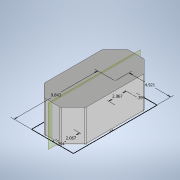
# Autodesk Inventor part: Bottle Holder
Saved by Autodesk Inventor 2020 (Build 240168000, 168)
## iProperties
Created: 2022-01-25
Part Number: Bottle Holder
Material: Generic
Document SubType Name: Modeling
Designer: Beaucage
Density: 1 g/cm^3
Appearance: Default
Author: Beaucage
Autodesk Inventor part; units mm, degrees
ref_plane "YZ Plane" through (0, 0, 0) normal (1, 0, 0) x (0, 1, 0)
ref_plane "XZ Plane" through (0, 0, 0) normal (0, 1, 0) x (-1, 0, 0)
ref_plane "XY Plane" through (0, 0, 0) normal (0, 0, 1) x (1, 0, 0)
sketch "Sketch1" plane through (0, 0, 0) normal (0, 1, 0) x (-1, 0, 0)
  line L0 (0, 0) -> (125, 0)
  line L1 (125, 0) -> (125, -250)
  line L2 (125, -250) -> (0, -250)
  line L3 (0, -250) -> (0, 0)
  line L4 (62.5, -250) -> (62.5, -240)
  line L5 (62.5, -240) -> (62.5, -187.5)
  line L6 (62.5, 0) -> (62.5, -10)
  line L7 (62.5, -10) -> (62.5, -62.5018)
  dimension "d0" = 125
  dimension "d1" = 250
  dimension "d2" = 10
  dimension "d3" = 52.5
  dimension "d4" = 10
  dimension "d5" = 52.5018
  constraints: 16 end point, 2 midpoint, 2 parallel, 2 point on line, 2 vertical, 1 horizontal, 1 perpendicular
  measures "d0" distance of L1.end L2.end
  measures "d1" distance of L0.end L1.end
  measures "d2" distance of L4.start L4.end
  measures "d3" distance of L4.end L5.end
  measures "d4" distance of L6.start L6.end
  measures "d5" distance of L6.end L7.end
extrude "Extrusion1" add sketch "Sketch1" along normal blind 100
hole "Hole1" at (-62.5, 0, -62.5018) at (-62.5, 0, -187.5) direction (0, 1, 0) diameter 105 depth 90
sketch "Sketch2" plane through (0, 0, 0) normal (0, -1, 0) x (1, 0, 0)
  line L0 (-125, -250) -> (-125, 0) projected
  line L1 (-125, -125) -> (-112.3, -125)
  line L2 (-112.3, -125) -> (-112.3, -121.825)
  line L3 (-112.3, -121.825) -> (-99.6, -121.825)
  line L4 (-99.6, -121.825) -> (-99.6, -128.175)
  line L5 (-99.6, -128.175) -> (-112.3, -128.175)
  line L6 (-112.3, -128.175) -> (-112.3, -121.825)
  line L7 (-112.3, -128.175) -> (-115.475, -128.175)
  line L8 (-115.475, -128.175) -> (-115.475, -121.825)
  line L9 (-115.475, -121.825) -> (-112.3, -121.825)
  line L10 (-112.3, -121.825) -> (-112.3, -128.175)
  point P0 (0, 0)
  dimension "d16" = 12.7
  dimension "d17" = 3.175
  dimension "d18" = 12.7
  dimension "d19" = 6.35
  dimension "d20" = 3.175
  constraints: 20 end point, 4 parallel, 3 horizontal, 3 perpendicular, 1 midpoint
  measures "d16" distance of L1.start L1.end
  measures "d17" distance of L1.end L2.end
  measures "d18" distance of L4.end L5.end
  measures "d19" distance of L3.end L4.end
  measures "d20" distance of L8.end L9.end
extrude "Extrusion2" add sketch "Sketch2" along normal blind 6.35 contours L8 L9 L2 L1 | L1 L6 L7 L8
sketch "Sketch3" plane through (0, -6.35, 0) normal (0, -1, 0) x (1, 0, 0)
  line L0 (-112.3, -128.175) -> (-112.3, -121.825) projected
  line L1 (-112.3, -121.825) -> (-99.6, -121.825)
  line L2 (-99.6, -121.825) -> (-99.6, -128.175)
  line L3 (-99.6, -128.175) -> (-112.3, -128.175)
  line L4 (-112.3, -128.175) -> (-112.3, -121.825)
  line L5 (-115.475, -128.175) -> (-115.475, -121.825) projected
  line L6 (-115.475, -121.825) -> (-112.3, -121.825)
  line L7 (-112.3, -121.825) -> (-112.3, -128.175)
  line L8 (-112.3, -128.175) -> (-115.475, -128.175)
  line L9 (-115.475, -128.175) -> (-115.475, -121.825)
  point P0 (0, 0)
  dimension "d23" = 12.7
  constraints: 16 end point, 4 parallel, 2 horizontal, 2 perpendicular
  measures "d23" distance of L2.end L3.end
extrude "Extrusion3" add sketch "Sketch3" along normal blind 3.175
fillet "Fillet2" radius 3.175 4 edges at (-115.475, 0, -125) (-113.8875, 0, -128.175) (-113.8875, 0, -121.825) (-112.3, 0, -125)
ref_plane "Work Plane1" through (-62.5, 0, -250) normal (-1, 0, 0) x (0, 0, 1)
mirror "Mirror1" about plane through (-62.5, 0, -250) normal (-1, 0, 0) of "Extrusion2", "Extrusion3", "Fillet2"
chamfer "Chamfer1" distance 38.1 angle 45 4 edges at (-125, 50, 0) (0, 50, 0) (0, 50, -250) (-125, 50, -250)
fillet "Fillet1" radius 6.35 16 edges at (-125, 0, -125) (-62.5, 0, 0) (0, 0, -125) (-62.5, 0, -250) (-105.95, 0, -19.05) (-19.05, 0, -19.05) (-19.05, 0, -230.95) (-105.95, 0, -230.95) (-125, 50, -38.1) (-86.9, 50, 0) (-38.1, 50, 0) (0, 50, -38.1) (0, 50, -211.9) (-86.9, 50, -250) (-125, 50, -211.9) (-38.1, 50, -250)
body "Solid1"
